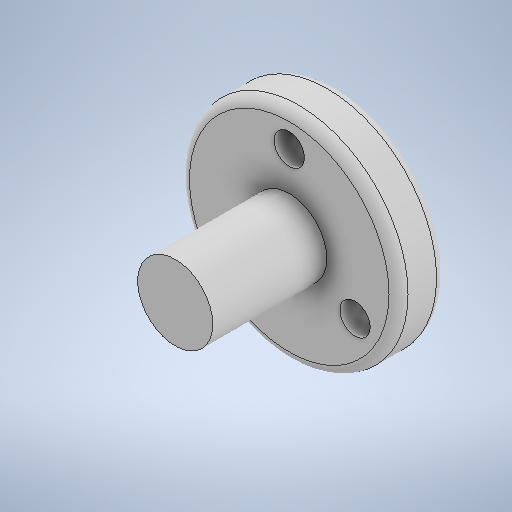
# Autodesk Inventor part: Eixo de suporte II
Saved by Autodesk Inventor 2025.2 (Build 292293000, 293)
## iProperties
Created: 2025-03-15
Part Number: Eixo de suporte II
Material: Generic
Document SubType Name: Modeling
Designer: erikg
Density: 1 g/cm^3
Appearance: Default
Author: erikg
Autodesk Inventor part; units mm, degrees
ref_plane "YZ Plane" through (0, 0, 0) normal (1, 0, 0) x (0, 1, 0)
ref_plane "XZ Plane" through (0, 0, 0) normal (0, 1, 0) x (-1, 0, 0)
ref_plane "XY Plane" through (0, 0, 0) normal (0, 0, 1) x (1, 0, 0)
sketch "Sketch1" plane through (0, 0, 0) normal (0, 0, 1) x (1, 0, 0)
  circle A0 centre (0, 0) radius 11.5
  dimension "d0" = 23
  constraints: 1 centre point, 1 coincident
  measures "d0" diameter of A0
extrude "Extrusion1" add sketch "Sketch1" along normal blind 5
sketch "Sketch2" plane through (0, 0, 5) normal (0, 0, 1) x (1, 0, 0)
  circle A0 centre (0, 0) radius 3.95
  dimension "d3" = 7.9
  constraints: 1 centre point, 1 coincident
  measures "d3" diameter of A0
extrude "Extrusion2" add sketch "Sketch2" along normal blind 12
sketch "Sketch3" plane through (0, 0, 0) normal (0, 0, -1) x (-1, 0, 0)
  circle A0 centre (0, 0) radius 4
  point P0 (0, 8)
  point P1 (-6.9282, -4)
  point P2 (6.9282, -4)
  dimension "d8" = 360
  dimension "d17" = 8
  constraints: 1 centre point, 1 coincident, 4 other
  measures "d17" distance of point (0, 0) point (0, 8)
hole "Hole1" at (0, 8, 0) at (6.9282, -4, 0) at (-6.9282, -4, 0) direction (0, 0, 1) diameter 3.2 end through all
fillet "Fillet1" radius 1 2 edges at (-11.5, 0, 0) (-11.5, 0, 5)
body "Solid1"
